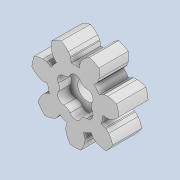
# Autodesk Inventor part: m2z7
Saved by Autodesk Inventor 2020.4 (Build 244396000, 396)
## iProperties
Created: 2021-04-23
Part Number: m2z7
Material: アルミニウム 2014-T4
Document SubType Name: Modeling
Designer: happy
Density: 2.8 g/cm^3
Appearance: サテン
Author: happy
Autodesk Inventor part; units mm, degrees
ref_plane "YZ Plane" through (0, 0, 0) normal (1, 0, 0) x (0, 1, 0)
ref_plane "XZ Plane" through (0, 0, 0) normal (0, 1, 0) x (-1, 0, 0)
ref_plane "XY Plane" through (0, 0, 0) normal (0, 0, 1) x (1, 0, 0)
sketch "スケッチ1" plane through (0, 0, 0) normal (0, 0, 1) x (1, 0, 0)
  arc A0 (149.5249, 111.6966) -> (149.4642, 111.5067) centre (150.3865, 111.3165) ccw
  arc A1 (149.9412, 112.3564) -> (149.5249, 111.6966) centre (151.9548, 110.6246) ccw
  arc A2 (151.4141, 113.5151) -> (149.9412, 112.3564) centre (153.6271, 109.1863) ccw
  arc A3 (143.9033, 109.9765) -> (144.0139, 109.8107) centre (144.7377, 110.4132) ccw
  arc A4 (143.647, 110.7134) -> (143.9033, 109.9765) centre (146.2564, 111.2079) ccw
  arc A5 (143.6595, 112.5874) -> (143.647, 110.7134) centre (148.4237, 111.6186) ccw
  arc A6 (141.7431, 104.509) -> (141.9418, 104.492) centre (141.922, 105.4335) ccw
  arc A7 (141.0072, 104.768) -> (141.7431, 104.509) centre (142.2475, 107.1165) ccw
  arc A8 (139.5499, 105.9462) -> (141.0072, 104.768) centre (143.2777, 109.0669) ccw
  arc A9 (144.671, 99.4111) -> (144.8081, 99.5559) centre (144.0597, 100.1274) ccw
  arc A10 (144.0096, 98.9973) -> (144.671, 99.4111) centre (142.9469, 101.4312) ccw
  arc A11 (142.1798, 98.5924) -> (144.0096, 98.9973) centre (142.0642, 103.4527) ccw
  arc A12 (150.4822, 98.5217) -> (150.4545, 98.7192) centre (149.541, 98.4903) ccw
  arc A13 (150.3933, 97.7466) -> (150.4822, 98.5217) centre (147.8278, 98.4333) ccw
  arc A14 (149.569, 96.0636) -> (150.3933, 97.7466) centre (145.697, 99.0035) ccw
  arc A15 (154.8007, 102.5106) -> (154.6291, 102.612) centre (154.2384, 101.7552) ccw
  arc A16 (155.3513, 101.9579) -> (154.8007, 102.5106) centre (153.2149, 100.3801) ccw
  arc A17 (156.1532, 100.264) -> (155.3513, 101.9579) centre (151.4405, 99.0698) ccw
  arc A18 (154.3747, 108.3739) -> (154.1884, 108.303) centre (154.6147, 107.4633) ccw
  arc A19 (155.1501, 108.4598) -> (154.3747, 108.3739) centre (155.0516, 105.8058) ccw
  arc A20 (156.9743, 108.0306) -> (155.1501, 108.4598) centre (154.9697, 103.6015) ccw
  arc A21 (147.5358, 111.5067) -> (147.4751, 111.6966) centre (146.6135, 111.3165) ccw
  arc A22 (147.4751, 111.6966) -> (147.0588, 112.3564) centre (145.0452, 110.6246) ccw
  arc A23 (147.0588, 112.3564) -> (145.5858, 113.5151) centre (143.3729, 109.1863) ccw
  arc A24 (142.8116, 108.303) -> (142.6253, 108.3739) centre (142.3853, 107.4633) ccw
  arc A25 (142.6253, 108.3739) -> (141.8499, 108.4598) centre (141.9484, 105.8058) ccw
  arc A26 (141.8499, 108.4598) -> (140.0256, 108.0306) centre (142.0302, 103.6015) ccw
  arc A27 (142.3709, 102.612) -> (142.1993, 102.5106) centre (142.7615, 101.7552) ccw
  arc A28 (142.1993, 102.5106) -> (141.6486, 101.9579) centre (143.7851, 100.3801) ccw
  arc A29 (141.6486, 101.9579) -> (140.8468, 100.264) centre (145.5595, 99.0698) ccw
  arc A30 (146.5455, 98.7192) -> (146.5178, 98.5217) centre (147.459, 98.4903) ccw
  arc A31 (146.5178, 98.5217) -> (146.6066, 97.7466) centre (149.1722, 98.4333) ccw
  arc A32 (146.6066, 97.7466) -> (147.431, 96.0636) centre (151.303, 99.0035) ccw
  arc A33 (152.1919, 99.5559) -> (152.329, 99.4111) centre (152.9403, 100.1274) ccw
  arc A34 (152.329, 99.4111) -> (152.9903, 98.9973) centre (154.0531, 101.4312) ccw
  arc A35 (152.9903, 98.9973) -> (154.8201, 98.5924) centre (154.9358, 103.4527) ccw
  arc A36 (155.0582, 104.492) -> (155.2568, 104.509) centre (155.078, 105.4335) ccw
  arc A37 (155.2568, 104.509) -> (155.9927, 104.768) centre (154.7524, 107.1165) ccw
  arc A38 (155.9927, 104.768) -> (157.4501, 105.9462) centre (153.7223, 109.0669) ccw
  arc A39 (152.986, 109.8107) -> (153.0967, 109.9765) centre (152.2623, 110.4132) ccw
  arc A40 (153.0967, 109.9765) -> (153.3529, 110.7134) centre (150.7435, 111.2079) ccw
  arc A41 (153.3529, 110.7134) -> (153.3404, 112.5874) centre (148.5763, 111.6186) ccw
  arc A42 (149.3355, 110.6383) -> (147.6645, 110.6383) centre (148.5, 104.9999) ccw
  arc A43 (144.6126, 109.1687) -> (143.5707, 107.8622) centre (148.5, 104.9999) ccw
  arc A44 (142.817, 104.5598) -> (143.1888, 102.9307) centre (148.5, 104.9999) ccw
  arc A45 (145.3008, 100.2824) -> (146.8063, 99.5573) centre (148.5, 104.9999) ccw
  arc A46 (150.1936, 99.5573) -> (151.6992, 100.2824) centre (148.5, 104.9999) ccw
  arc A47 (153.8111, 102.9307) -> (154.183, 104.5598) centre (148.5, 104.9999) ccw
  arc A48 (153.4292, 107.8622) -> (152.3873, 109.1687) centre (148.5, 104.9999) ccw
  arc A49 (145.5858, 113.5151) -> (143.6595, 112.5874) centre (148.5, 104.9999) ccw
  arc A50 (140.0256, 108.0306) -> (139.5499, 105.9462) centre (148.5, 104.9999) ccw
  arc A51 (140.8468, 100.264) -> (142.1798, 98.5924) centre (148.5, 104.9999) ccw
  arc A52 (147.431, 96.0636) -> (149.569, 96.0636) centre (148.5, 104.9999) ccw
  arc A53 (154.8201, 98.5924) -> (156.1532, 100.264) centre (148.5, 104.9999) ccw
  arc A54 (157.4501, 105.9462) -> (156.9743, 108.0306) centre (148.5, 104.9999) ccw
  arc A55 (153.3404, 112.5874) -> (151.4141, 113.5151) centre (148.5, 104.9999) ccw
  line L0 (149.3355, 110.6383) -> (149.4642, 111.5067)
  line L1 (144.6126, 109.1687) -> (144.0139, 109.8107)
  line L2 (142.817, 104.5598) -> (141.9418, 104.492)
  line L3 (145.3008, 100.2824) -> (144.8081, 99.5559)
  line L4 (150.1936, 99.5573) -> (150.4545, 98.7192)
  line L5 (153.8111, 102.9307) -> (154.6291, 102.612)
  line L6 (153.4292, 107.8622) -> (154.1884, 108.303)
  line L7 (147.6645, 110.6383) -> (147.5358, 111.5067)
  line L8 (143.5707, 107.8622) -> (142.8116, 108.303)
  line L9 (143.1888, 102.9307) -> (142.3709, 102.612)
  line L10 (146.8063, 99.5573) -> (146.5455, 98.7192)
  line L11 (151.6992, 100.2824) -> (152.1919, 99.5559)
  line L12 (154.183, 104.5598) -> (155.0582, 104.492)
  line L13 (152.3873, 109.1687) -> (152.986, 109.8107)
  line L14 (137.5, 105) -> (159.5, 105)
  line L15 (148.5, 94) -> (148.5, 116)
  line L16 (177.5, 113.9999) -> (247.5, 113.9999)
  line L17 (177.5, 105.9999) -> (247.5, 105.9999)
  line L18 (177.5, 97.9999) -> (247.5, 97.9999)
  line L19 (177.5, 89.9999) -> (247.5, 89.9999)
  line L20 (177.5, 81.9999) -> (247.5, 81.9999)
  line L21 (177.5, 73.9999) -> (247.5, 73.9999)
  line L22 (177.5, 65.9999) -> (247.5, 65.9999)
  line L23 (177.5, 57.9999) -> (247.5, 57.9999)
  line L24 (177.5, 49.9999) -> (247.5, 49.9999)
  line L25 (177.5, 41.9999) -> (247.5, 41.9999)
  line L26 (177.5, 33.9999) -> (247.5, 33.9999)
  line L27 (177.5, 25.9999) -> (247.5, 25.9999)
  line L28 (177.5, 17.9999) -> (247.5, 17.9999)
  line L29 (177.5, 113.9999) -> (177.5, 17.9999)
  line L30 (247.5, 113.9999) -> (247.5, 17.9999)
  line L31 (212.5, 105.9999) -> (212.5, 17.9999)
  arc A56 (151.9641, 105.75) -> (150.8816, 107.625) centre (150.8816, 106.375) ccw
  arc A57 (151.9641, 105.75) -> (151.9641, 104.25) centre (153.2631, 105) ccw
  arc A58 (150.8816, 102.375) -> (151.9641, 104.25) centre (150.8816, 103.625) ccw
  arc A59 (147.4175, 101.625) -> (149.5825, 101.625) centre (148.5, 102.25) ccw
  arc A60 (150.8816, 102.375) -> (149.5825, 101.625) centre (150.8816, 100.875) ccw
  arc A61 (147.4175, 101.625) -> (146.1184, 102.375) centre (146.1184, 100.875) ccw
  arc A62 (146.1184, 107.625) -> (145.0359, 105.75) centre (146.1184, 106.375) ccw
  arc A63 (146.1184, 107.625) -> (147.4175, 108.375) centre (146.1184, 109.125) ccw
  line L32 (145.0359, 107) -> (148.5, 109) construction
  circle A64 centre (148.5, 105) radius 5 construction
  arc A65 (149.5825, 108.375) -> (147.4175, 108.375) centre (148.5, 107.75) ccw
  arc A66 (145.0359, 104.25) -> (145.0359, 105.75) centre (143.7369, 105) ccw
  arc A67 (149.5825, 108.375) -> (150.8816, 107.625) centre (150.8816, 109.125) ccw
  line L33 (145.0359, 103) -> (145.0359, 107) construction
  arc A68 (145.0359, 104.25) -> (146.1184, 102.375) centre (146.1184, 103.625) ccw
  line L34 (148.5, 109) -> (151.9641, 107) construction
  line L35 (148.5, 101) -> (145.0359, 103) construction
  circle A69 centre (148.5, 105) radius 4 construction
  circle A70 centre (148.5, 105) radius 3.2631 construction
  line L36 (151.9641, 103) -> (148.5, 101) construction
  line L37 (151.9641, 107) -> (151.9641, 103) construction
  circle A71 centre (148.5, 105) radius 2.025
  point P0 (0, 0)
  point P1 (183.5, 108)
  point P2 (186, 100)
  point P3 (186, 92)
  point P4 (183.5, 84)
  point P5 (186, 76)
  point P6 (181, 68)
  point P7 (183.5, 60)
  point P8 (183.5, 52)
  point P9 (183.5, 44)
  point P10 (186, 36)
  point P11 (186, 28)
  point P12 (183.5, 20)
  point P13 (213.5, 100)
  point P14 (229.75, 92)
  point P15 (229.75, 84)
  point P16 (226, 76)
  point P17 (228.5, 68)
  point P18 (222.25, 60)
  point P19 (228.5, 52)
  point P20 (226, 44)
  point P21 (223.5, 36)
  point P22 (231, 28)
  point P23 (231, 20)
  point P24 (149.5, 129.5)
  point P25 (149.5, 123.5)
  point P26 (166.75, 129.5)
  point P27 (168.875, 123.5)
  point P28 (151.9641, 107)
  point P29 (151.9641, 103)
  point P30 (148.5, 101)
  point P31 (145.0359, 103)
  point P32 (151.9641, 105.75)
  point P33 (151.9641, 104.25)
  point P34 (150.8816, 102.375)
  point P35 (149.5825, 101.625)
  point P36 (147.4175, 101.625)
  point P37 (146.1184, 102.375)
  point P38 (145.0359, 104.25)
  point P39 (145.0359, 105.75)
  point P40 (146.1184, 107.625)
  dimension "d5" = 8
  dimension "d4" = 10
  dimension "d6" = 360
  dimension "d7" = 360
  dimension "d8" = 6.5263
  dimension "d9" = 1.5
  dimension "d10" = 1.25
  dimension "d11" = 4.05
  constraints: 142 point on circle, 72 end point, 71 centre point, 39 equal radius, 37 tangent, 13 parallel, 6 concentric, 5 coincident, 3 horizontal, 3 midpoint, 2 perpendicular, 2 point on line, 2 vertical, 1 vertical alignment, 313 other
  measures "d4" diameter of A64
  measures "d8" diameter of A70
  measures "d9" radius of A67
  measures "d10" radius of A65
  measures "d11" diameter of A71
extrude "押し出し1" add sketch "スケッチ1" along normal blind 6 contours A1 A2 A55 A41 A40 A39 L13 A48 L6 A18 A19 A20 A54 A38 L14 A57 A56 A67 A65 L15 A42 L0 A0 | L15 A65 A63 A62 A66 L14 A8 A50 A26 A25 A24 L8 A43 L1 A3 A4 A5 A49 A23 A22 A21 L7 A42 | L14 A38 A37 A36 L12 A47 L5 A15 A16 A17 A53 A35 A34 A33 L11 A46 L4 A12 A13 A14 A52 L15 A59 A60 A58 A57 | A66 A68 A61 A59 L15 A52 A32 A31 A30 L10 A45 L3 A9 A10 A11 A51 A29 A28 A27 L9 A44 L2 A6 A7 A8 L14
extrude "押し出し2" add sketch "スケッチ1" along normal blind 3.5 contours A65 A67 A56 A57 L14 A71 L15 | L15 A71 L14 A66 A62 A63 A65 | L14 A57 A58 A60 A59 L15 A71 | A71 L15 A59 A61 A68 A66 L14
